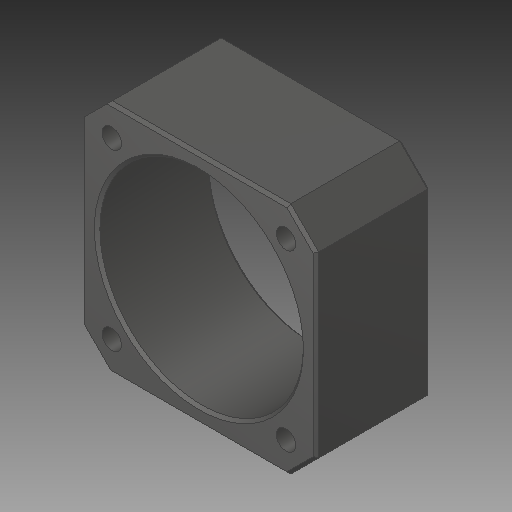
# Autodesk Inventor part: Cache reducteur
Saved by Autodesk Inventor 2017 (Build 210142000, 142)
## iProperties
Company: FABLAB Frenchmakers
Part Number: Cache reducteur
Material: ----------
Document SubType Name: Modeling
Designer: FABLAB Frenchmakers
Density: 7.86 g/cm^3
Appearance: Aluminium - Plat(1)
Mass: 100.852 g
Surface Area: 75.5765 cm^2
Volume: 12.831 cm^3
Project: 1420 Vauban 3D XL
Catalog Web Link: http://frenchmakers.com/
Stock Number: 1420-05-12
Autodesk Inventor part; units mm, degrees
ref_plane "YZ Plane" through (0, 0, 0) normal (1, 0, 0) x (0, 1, 0)
ref_plane "XZ Plane" through (0, 0, 0) normal (0, 1, 0) x (-1, 0, 0)
ref_plane "XY Plane" through (0, 0, 0) normal (0, 0, 1) x (1, 0, 0)
sketch "Esquisse1" plane through (0, 0, 0) normal (0, 0, 1) x (1, 0, 0)
  line L0 (-21, -21) -> (21, -21)
  line L1 (21, -21) -> (21, 21)
  line L2 (21, 21) -> (-21, 21)
  line L3 (-21, 21) -> (-21, -21)
  line L4 (-21, -21) -> (21, 21) construction
  line L5 (21, -21) -> (-21, 21) construction
  point P0 (0, 0)
  dimension "d0" = 42
  dimension "d1" = 42
  constraints: 12 end point, 2 midpoint, 2 parallel, 1 horizontal, 1 perpendicular
  measures "d0" distance between parallel lines of L1 L3
  measures "d1" distance between parallel lines of L0 L2
extrude "Extrusion1" add sketch "Esquisse1" along normal mid plane 20.5
sketch "Esquisse2" plane through (0, 0, 10.25) normal (0, 0, 1) x (1, 0, 0)
  point P0 (0, 0)
  point P1 (0, 0)
  constraints: 1 coincident
hole "Perçage1" at (0, 0, 10.25) direction (0, 0, -1) diameter 36.5 end through all
sketch "Esquisse3" plane through (0, 0, 10.25) normal (0, 0, 1) x (1, 0, 0)
  point P0 (0, 0)
  point P1 (-15.625, 15.625)
  point P2 (-15.625, -15.625)
  point P3 (15.625, -15.625)
  point P4 (15.625, 15.625)
  dimension "d11" = 31.25
  dimension "d12" = 31.25
  dimension "d13" = 15.625
  dimension "d14" = 15.625
  constraints: 2 horizontal alignment, 2 vertical alignment
  measures "d11" distance of point (15.625, 15.625) point (-15.625, 15.625)
  measures "d12" distance of point (15.625, -15.625) point (15.625, 15.625)
  measures "d13" horizontal distance of point (0, 0) point (15.625, 15.625)
  measures "d14" horizontal distance of point (0, 0) point (15.625, 15.625)
hole "Perçage2" at (-15.625, 15.625, 10.25) at (-15.625, -15.625, 10.25) at (15.625, -15.625, 10.25) at (15.625, 15.625, 10.25) direction (0, 0, -1) diameter 3.5 end through all
chamfer "Chanfrein1" distance 5 angle 45 4 edges at (21, 21, 0) (-21, 21, 0) (21, -21, 0) (-21, -21, 0)
chamfer "Chanfrein2" distance 0.5 angle 45 17 edges at (-21, 0, 10.25) (-18.5, -18.5, 10.25) (0, -21, 10.25) (18.5, -18.5, 10.25) (21, 0, 10.25) (18.5, 18.5, 10.25) (0, 21, 10.25) (0, 18.25, 10.25) (-18.5, 18.5, -10.25) (0, 21, -10.25) (0, 18.25, -10.25) (-21, 0, -10.25) (0, -21, -10.25) (-18.5, -18.5, -10.25) (18.5, -18.5, -10.25) (21, 0, -10.25) (18.5, 18.5, -10.25)
equation "\"d12\" = d11"
equation "\"d13\" = 0.5 * d11"
equation "\"d14\" = 0.5 * d12"
